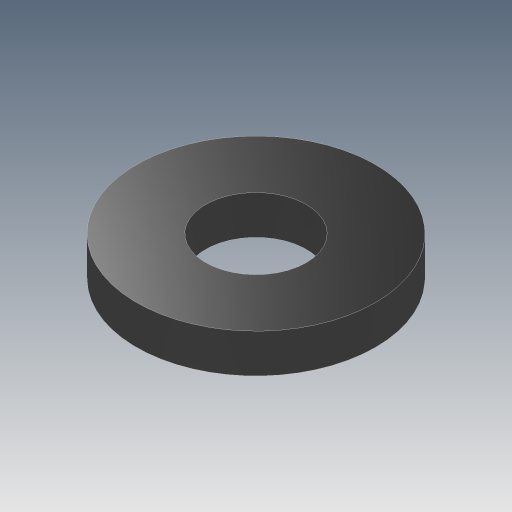
# Autodesk Inventor part: Plastic Washer (RAM-201U-B)
Saved by Autodesk Inventor 2023.1 (Build 271208000, 208)
## iProperties
Created: 2023-01-24
Part Number: Plastic Washer (RAM-201U-B)
Material: Plastica PPS
Document SubType Name: Modeling
Designer: Cominelli Nicolas
Mass: 1.31326 g
Surface Area: 7.82885 cm^2
Volume: 0.802237 cm^3
Density: 1.637 g/cm^3
Appearance: Lucida - Nero
Author: Cominelli Nicolas
Costo: 0
Trattamento: -
Autodesk Inventor part; units mm, degrees
ref_plane "YZ Plane" through (0, 0, 0) normal (1, 0, 0) x (0, 1, 0)
ref_plane "XZ Plane" through (0, 0, 0) normal (0, 1, 0) x (-1, 0, 0)
ref_plane "XY Plane" through (0, 0, 0) normal (0, 0, 1) x (1, 0, 0)
sketch "Schizzo4" plane through (0, 0, 0) normal (0, 0, 1) x (1, 0, 0)
  line L0 (4.15, 0) -> (4.15, 3.2)
  line L1 (4.15, 3.2) -> (9.85, 3.2)
  line L2 (9.85, 3.2) -> (9.85, 0)
  line L3 (9.85, 0) -> (4.15, 0)
  line L4 (0, 0) -> (0, 3.2)
  dimension "d0" = 3.2
  dimension "d1" = 19.7
  dimension "d2" = 8.3
  constraints: 10 end point, 3 perpendicular, 2 vertical, 1 horizontal alignment
  measures "d0" distance of L1.end L2.end
  measures "d1" diameter of L2 L4
  measures "d2" diameter of L0 L4
revolve "Rivoluzione1" add sketch "Schizzo4" angle 360 about axis through (0, 0, 0) along (0, 1, 0)
